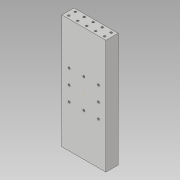
# Autodesk Inventor part: dynamixel_pro_frame_part1
Saved by Autodesk Inventor 2017 (Build 210142000, 142)
## iProperties
Part Number: dynamixel_pro_frame_part1
Material: Aluminium 6061
Document SubType Name: Modeling
Designer: Max
Density: 2.7 g/cm^3
Appearance: Vorgabe
Mass: 108.385 g
Surface Area: 257.694 cm^2
Volume: 40.1425 cm^3
Author: Max
Autodesk Inventor part; units mm, degrees
ref_plane "YZ Plane" through (0, 0, 0) normal (1, 0, 0) x (0, 1, 0)
ref_plane "XZ Plane" through (0, 0, 0) normal (0, 1, 0) x (-1, 0, 0)
ref_plane "XY Plane" through (0, 0, 0) normal (0, 0, 1) x (1, 0, 0)
sketch "Skizze1" plane through (0, 0, 0) normal (0, 1, 0) x (-1, 0, 0)
  line L0 (-27, 70) -> (27, 70)
  line L1 (27, 70) -> (27, -70)
  line L2 (27, -70) -> (-27, -70)
  line L3 (-27, -70) -> (-27, 70)
  line L4 (-27, 70) -> (27, -70) construction
  line L5 (27, 70) -> (-27, -70) construction
  point P0 (0, 0)
  dimension "d0" = 54
  dimension "d1" = 140
  constraints: 12 end point, 2 midpoint, 2 parallel, 1 horizontal, 1 perpendicular
  measures "d0" distance of L1.end L2.end
  measures "d1" distance of L0.end L1.end
extrude "Extrusion1" add sketch "Skizze1" along normal blind 15
sketch "Skizze2" plane through (0, 15, 0) normal (0, 1, 0) x (1, 0, 0)
  line L0 (24, -63) -> (-24, -63)
  line L1 (-24, -63) -> (-24, 63)
  line L2 (-24, 63) -> (24, 63)
  line L3 (24, 63) -> (24, -63)
  line L4 (24, -63) -> (-24, 63) construction
  line L5 (-24, -63) -> (24, 63) construction
  line L6 (-27, -70) -> (27, -70) projected
  line L7 (27, -70) -> (27, 70) projected
  line L8 (27, 70) -> (-27, 70) projected
  line L9 (-27, 70) -> (-27, -70) projected
  point P0 (0, 0)
  dimension "d4" = 3
  dimension "d7" = 7
  constraints: 12 end point, 2 midpoint, 2 parallel, 1 horizontal, 1 perpendicular
  measures "d4" distance between parallel lines of L9 L1
  measures "d7" distance between parallel lines of L8 L2
extrude "Extrusion2" cut sketch "Skizze2" against normal blind 12 contours L0 L1 L2 L3
sketch "Skizze4" plane through (-27, 0, 70) normal (0, 0, 1) x (1, 0, 0)
  line L0 (54, 0) -> (0, 0) projected
  line L1 (54, 0) -> (54, 15) projected
  line L2 (0, 15) -> (54, 15) projected
  line L3 (0, 0) -> (0, 15) projected
  point P0 (27, 3.5)
  dimension "d23" = 3.5
  measures "d23" distance from line of L0 point (27, 3.5)
hole "Bohrung1" at (0, 3.5, 70) direction (0, 0, -1) diameter 2.459 depth 5 tip angle 118 thread size "M3x0.5" class "6H" standard "ISO Metric profile"
pattern_linear "Rechteckige Anordnung1" count 5 spacing 11 along (-1, 0, 0) count 2 spacing 8 along (0, 1, 0) of "Bohrung1" first direction both ways yes
mirror "Spiegeln1" about plane through (0, 0, 0) normal (0, 0, 1) of "Extrusion2", "Bohrung1", "Rechteckige Anordnung1"
sketch "Skizze6" plane through (0, 0, 0) normal (0, -1, 0) x (1, 0, 0)
  line L0 (-18, 18) -> (18, 18)
  line L1 (18, 18) -> (18, -18)
  line L2 (18, -18) -> (-18, -18)
  line L3 (-18, -18) -> (-18, 18)
  line L4 (-18, 18) -> (18, -18) construction
  line L5 (18, 18) -> (-18, -18) construction
  line L6 (0, 18) -> (0, -18) construction
  line L7 (-18, 0) -> (18, 0) construction
  point P0 (0, 0)
  dimension "d47" = 36
  dimension "d48" = 36
  constraints: 16 end point, 6 midpoint, 2 parallel, 1 horizontal, 1 perpendicular
  measures "d47" distance of L0.end L1.end
  measures "d48" distance of L1.end L2.end
hole "Bohrung2" at (18, 0, 18) at (18, 0, 0) at (18, 0, -18) at (0, 0, -18) at (-18, 0, -18) at (-18, 0, 0) at (-18, 0, 18) at (0, 0, 18) direction (0, 1, 0) diameter 2.459 depth 8.8 tip angle 118 thread size "M3x0.5" class "6H" standard "ISO Metric profile"
fillet "Rundung2" radius 4 4 edges at (-24, 9, -63) (24, 9, -63) (24, 9, 63) (-24, 9, 63)
